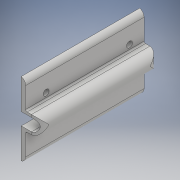
# Autodesk Inventor part: Part1
Saved by Autodesk Inventor 2018.3 (Build 223285000, 285)
## iProperties
Created: 2021-05-17
Part Number: Part1
Material: Generic
Document SubType Name: Modeling
Designer: Eugene
Density: 1 g/cm^3
Appearance: Default
Author: Eugene
Autodesk Inventor part; units mm, degrees
ref_plane "YZ Plane" through (0, 0, 0) normal (1, 0, 0) x (0, 1, 0)
ref_plane "XZ Plane" through (0, 0, 0) normal (0, 1, 0) x (-1, 0, 0)
ref_plane "XY Plane" through (0, 0, 0) normal (0, 0, 1) x (1, 0, 0)
sketch "Sketch1" plane through (0, 0, 0) normal (1, 0, 0) x (0, 1, 0)
  line L0 (0, 0) -> (81, 0)
  line L1 (81, 0) -> (81, -50)
  line L2 (81, -50) -> (0, -50)
  line L3 (0, -50) -> (0, 0)
  circle A0 centre (71, -15) radius 2
  circle A1 centre (71, -34) radius 2
  circle A2 centre (14, -15) radius 2
  circle A3 centre (14, -34) radius 2
  dimension "d0" = 81
  dimension "d1" = 50
  dimension "d2" = 4
  dimension "d3" = 15
  dimension "d4" = 4
  dimension "d5" = 16
  dimension "d6" = 4
  dimension "d7" = 15
  dimension "d8" = 4
  dimension "d9" = 57
  dimension "d11" = 10
  dimension "d12" = 57
  dimension "d13" = 10
  constraints: 8 end point, 4 centre point, 2 parallel, 1 horizontal, 1 perpendicular
  measures "d0" distance of L1.end L2.end
  measures "d1" distance of L0.end L1.end
  measures "d2" diameter of A0
  measures "d3" distance from line of L0 A0.centre
  measures "d4" diameter of A1
  measures "d5" distance from line of L2 A1.centre
  measures "d6" diameter of A2
  measures "d7" distance from line of L0 A2.centre
  measures "d8" diameter of A3
  measures "d9" distance of A3.centre A1.centre
  measures "d11" distance from line of L1 A1.centre
  measures "d12" distance of A2.centre A0.centre
  measures "d13" distance from line of L1 A0.centre
extrude "Extrusion1" add sketch "Sketch1" along normal blind 3
sketch "Sketch5" plane through (0, 81, 0) normal (0, 1, 0) x (1, 0, 0)
  circle A0 centre (7, 25) radius 4
  line L0 (0, 0) -> (3, 0) projected
  line L1 (3, 50) -> (3, 0) projected
  dimension "d26" = 8
  dimension "d27" = 25
  dimension "d28" = 4
  constraints: 1 centre point
  measures "d26" diameter of A0
  measures "d27" distance from line of L0 A0.centre
  measures "d28" distance from line of L1 A0.centre
extrude "Extrusion3" add sketch "Sketch5" against normal blind 81
sketch "Sketch9" plane through (7, 81, -25) normal (0, 1, 0) x (1, 0, 0)
  line L0 (-4, 0) -> (-4, -25) projected
  line L1 (-4, -6) -> (6, -6)
  line L2 (6, -6) -> (6, 6)
  line L3 (6, 6) -> (-4, 6)
  line L4 (-4, 6) -> (-4, -6)
  line L5 (-7, -25) -> (-4, -25) projected
  dimension "d42" = 10
  dimension "d43" = 12
  dimension "d44" = 19
  constraints: 8 end point, 2 parallel, 1 horizontal, 1 perpendicular, 1 point on line
  measures "d42" distance of L3.end L2.end
  measures "d43" distance of L2.end L1.end
  measures "d44" distance between parallel lines of L5 L1
extrude "Extrusion6" add sketch "Sketch9" against normal blind 81
sketch "Sketch10" plane through (0, 81, 0) normal (0, 1, 0) x (1, 0, 0)
  line L0 (3, 19) -> (13, 19) projected
  line L1 (13, 19) -> (13, 31) projected
  line L2 (7, 29.25) -> (0, 29.25)
  line L3 (0, 50) -> (0, 0) projected
  line L4 (7, 20.75) -> (0, 20.75)
  arc A0 (7, 20.75) -> (7, 29.25) centre (7, 25) ccw
  arc A1 (7, 20.75) -> (7, 29.25) centre (7, 25) ccw
  arc A2 (7, 20.75) -> (7, 29.25) centre (7, 25) ccw
  dimension "d55" = 4.25
  dimension "d56" = 4.25
  dimension "d57" = 4.25
  constraints: 6 point on circle, 4 end point, 3 centre point, 2 point on line, 1 horizontal, 1 parallel
  measures "d55" radius of A0
  measures "d56" radius of A1
  measures "d57" radius of A2
extrude "Extrusion8" cut sketch "Sketch10" against normal blind 81
fillet "Fillet4" radius 4 2 edges at (3, 40.5, 0) (3, 40.5, -50)
fillet "Fillet5" radius 1 2 edges at (3, 40.5, -19) (3, 40.5, -31)
fillet "Fillet6" radius 6 4 edges at (13, 81, -25) (13, 0, -25) (13, 40.5, -19) (13, 40.5, -31)
body "Solid1"
